Autodesk Fusion 360 part; units mm, degrees
(part 14 of 14)
  line L10014 (-7.2618, 368.3) -> (-12.7611, 377.825)
  line L10015 (-12.7611, 358.775) -> (-7.2618, 368.3)
  line L10016 (6.4863, 388.9375) -> (-4.5122, 388.9375)
  line L10017 (-4.5122, 388.9375) -> (-10.0114, 379.4125)
  line L10018 (-10.0114, 379.4125) -> (-4.5122, 369.8875)
  line L10019 (-4.5122, 369.8875) -> (6.4863, 369.8875)
  line L10020 (11.9856, 379.4125) -> (6.4863, 388.9375)
  line L10021 (6.4863, 369.8875) -> (11.9856, 379.4125)
  line L10022 (25.7337, 400.05) -> (14.7352, 400.05)
  line L10023 (14.7352, 400.05) -> (9.236, 390.525)
  line L10024 (9.236, 390.525) -> (14.7352, 381)
  line L10025 (14.7352, 381) -> (25.7337, 381)
  line L10026 (31.233, 390.525) -> (25.7337, 400.05)
  line L10027 (25.7337, 381) -> (31.233, 390.525)
  line L10028 (44.9812, 411.1625) -> (33.9826, 411.1625)
  line L10029 (33.9826, 411.1625) -> (28.4834, 401.6375)
  line L10030 (28.4834, 401.6375) -> (33.9826, 392.1125)
  line L10031 (33.9826, 392.1125) -> (44.9812, 392.1125)
  line L10032 (50.4804, 401.6375) -> (44.9812, 411.1625)
  line L10033 (44.9812, 392.1125) -> (50.4804, 401.6375)
  line L10034 (64.2286, 422.275) -> (53.2301, 422.275)
  line L10035 (53.2301, 422.275) -> (47.7308, 412.75)
  line L10036 (47.7308, 412.75) -> (53.2301, 403.225)
  line L10037 (53.2301, 403.225) -> (64.2286, 403.225)
  line L10038 (69.7278, 412.75) -> (64.2286, 422.275)
  line L10039 (64.2286, 403.225) -> (69.7278, 412.75)
  line L10040 (83.476, 433.3875) -> (72.4775, 433.3875)
  line L10041 (72.4775, 433.3875) -> (66.9782, 423.8625)
  line L10042 (66.9782, 423.8625) -> (72.4775, 414.3375)
  line L10043 (72.4775, 414.3375) -> (83.476, 414.3375)
  line L10044 (88.9753, 423.8625) -> (83.476, 433.3875)
  line L10045 (83.476, 414.3375) -> (88.9753, 423.8625)
  line L10046 (102.7234, 444.5) -> (91.7249, 444.5)
  line L10047 (91.7249, 444.5) -> (86.2256, 434.975)
  line L10048 (86.2256, 434.975) -> (91.7249, 425.45)
  line L10049 (91.7249, 425.45) -> (102.7234, 425.45)
  line L10050 (108.2227, 434.975) -> (102.7234, 444.5)
  line L10051 (102.7234, 425.45) -> (108.2227, 434.975)
  line L10052 (121.9708, 455.6125) -> (110.9723, 455.6125)
  line L10053 (110.9723, 455.6125) -> (105.473, 446.0875)
  line L10054 (105.473, 446.0875) -> (110.9723, 436.5625)
  line L10055 (110.9723, 436.5625) -> (121.9708, 436.5625)
  line L10056 (127.4701, 446.0875) -> (121.9708, 455.6125)
  line L10057 (121.9708, 436.5625) -> (127.4701, 446.0875)
  line L10058 (141.2182, 466.725) -> (130.2197, 466.725)
  line L10059 (130.2197, 466.725) -> (124.7205, 457.2)
  line L10060 (124.7205, 457.2) -> (130.2197, 447.675)
  line L10061 (130.2197, 447.675) -> (141.2182, 447.675)
  line L10062 (146.7175, 457.2) -> (141.2182, 466.725)
  line L10063 (141.2182, 447.675) -> (146.7175, 457.2)
  line L10064 (160.4657, 477.8375) -> (149.4671, 477.8375)
  line L10065 (149.4671, 477.8375) -> (143.9679, 468.3125)
  line L10066 (143.9679, 468.3125) -> (149.4671, 458.7875)
  line L10067 (149.4671, 458.7875) -> (160.4657, 458.7875)
  line L10068 (165.9649, 468.3125) -> (160.4657, 477.8375)
  line L10069 (160.4657, 458.7875) -> (165.9649, 468.3125)
  line L10070 (179.7131, 488.95) -> (168.7145, 488.95)
  line L10071 (168.7145, 488.95) -> (163.2153, 479.425)
  line L10072 (163.2153, 479.425) -> (168.7145, 469.9)
  line L10073 (168.7145, 469.9) -> (179.7131, 469.9)
  line L10074 (185.2123, 479.425) -> (179.7131, 488.95)
  line L10075 (179.7131, 469.9) -> (185.2123, 479.425)
  line L10076 (198.9605, 500.0625) -> (187.962, 500.0625)
  line L10077 (187.962, 500.0625) -> (182.4627, 490.5375)
  line L10078 (182.4627, 490.5375) -> (187.962, 481.0125)
  line L10079 (187.962, 481.0125) -> (198.9605, 481.0125)
  line L10080 (204.4597, 490.5375) -> (198.9605, 500.0625)
  line L10081 (198.9605, 481.0125) -> (204.4597, 490.5375)
  line L10082 (218.2079, 511.175) -> (207.2094, 511.175)
  line L10083 (207.2094, 511.175) -> (201.7101, 501.65)
  line L10084 (201.7101, 501.65) -> (207.2094, 492.125)
  line L10085 (207.2094, 492.125) -> (218.2079, 492.125)
  line L10086 (223.7072, 501.65) -> (218.2079, 511.175)
  line L10087 (218.2079, 492.125) -> (223.7072, 501.65)
  line L10088 (237.4553, 522.2875) -> (226.4568, 522.2875)
  line L10089 (226.4568, 522.2875) -> (220.9575, 512.7625)
  line L10090 (220.9575, 512.7625) -> (226.4568, 503.2375)
  line L10091 (226.4568, 503.2375) -> (237.4553, 503.2375)
  line L10092 (242.9546, 512.7625) -> (237.4553, 522.2875)
  line L10093 (237.4553, 503.2375) -> (242.9546, 512.7625)
  line L10094 (-917.3896, -122.2375) -> (-928.3881, -122.2375)
  line L10095 (-928.3881, -122.2375) -> (-933.8874, -131.7625)
  line L10096 (-933.8874, -131.7625) -> (-928.3881, -141.2875)
  line L10097 (-928.3881, -141.2875) -> (-917.3896, -141.2875)
  line L10098 (-911.8903, -131.7625) -> (-917.3896, -122.2375)
  line L10099 (-917.3896, -141.2875) -> (-911.8903, -131.7625)
  line L10100 (-898.1422, -111.125) -> (-909.1407, -111.125)
  line L10101 (-909.1407, -111.125) -> (-914.6399, -120.65)
  line L10102 (-914.6399, -120.65) -> (-909.1407, -130.175)
  line L10103 (-909.1407, -130.175) -> (-898.1422, -130.175)
  line L10104 (-892.6429, -120.65) -> (-898.1422, -111.125)
  line L10105 (-898.1422, -130.175) -> (-892.6429, -120.65)
  line L10106 (-878.8947, -100.0125) -> (-889.8933, -100.0125)
  line L10107 (-889.8933, -100.0125) -> (-895.3925, -109.5375)
  line L10108 (-895.3925, -109.5375) -> (-889.8933, -119.0625)
  line L10109 (-889.8933, -119.0625) -> (-878.8947, -119.0625)
  line L10110 (-873.3955, -109.5375) -> (-878.8947, -100.0125)
  line L10111 (-878.8947, -119.0625) -> (-873.3955, -109.5375)
  line L10112 (-859.6473, -88.9) -> (-870.6458, -88.9)
  line L10113 (-870.6458, -88.9) -> (-876.1451, -98.425)
  line L10114 (-876.1451, -98.425) -> (-870.6458, -107.95)
  line L10115 (-870.6458, -107.95) -> (-859.6473, -107.95)
  line L10116 (-854.1481, -98.425) -> (-859.6473, -88.9)
  line L10117 (-859.6473, -107.95) -> (-854.1481, -98.425)
  line L10118 (-840.3999, -77.7875) -> (-851.3984, -77.7875)
  line L10119 (-851.3984, -77.7875) -> (-856.8977, -87.3125)
  line L10120 (-856.8977, -87.3125) -> (-851.3984, -96.8375)
  line L10121 (-851.3984, -96.8375) -> (-840.3999, -96.8375)
  line L10122 (-834.9006, -87.3125) -> (-840.3999, -77.7875)
  line L10123 (-840.3999, -96.8375) -> (-834.9006, -87.3125)
  line L10124 (-821.1525, -66.675) -> (-832.151, -66.675)
  line L10125 (-832.151, -66.675) -> (-837.6503, -76.2)
  line L10126 (-837.6503, -76.2) -> (-832.151, -85.725)
  line L10127 (-832.151, -85.725) -> (-821.1525, -85.725)
  line L10128 (-815.6532, -76.2) -> (-821.1525, -66.675)
  line L10129 (-821.1525, -85.725) -> (-815.6532, -76.2)
  line L10130 (-801.9051, -55.5625) -> (-812.9036, -55.5625)
  line L10131 (-812.9036, -55.5625) -> (-818.4029, -65.0875)
  line L10132 (-818.4029, -65.0875) -> (-812.9036, -74.6125)
  line L10133 (-812.9036, -74.6125) -> (-801.9051, -74.6125)
  line L10134 (-796.4058, -65.0875) -> (-801.9051, -55.5625)
  line L10135 (-801.9051, -74.6125) -> (-796.4058, -65.0875)
  line L10136 (-782.6577, -44.45) -> (-793.6562, -44.45)
  line L10137 (-793.6562, -44.45) -> (-799.1554, -53.975)
  line L10138 (-799.1554, -53.975) -> (-793.6562, -63.5)
  line L10139 (-793.6562, -63.5) -> (-782.6577, -63.5)
  line L10140 (-777.1584, -53.975) -> (-782.6577, -44.45)
  line L10141 (-782.6577, -63.5) -> (-777.1584, -53.975)
  line L10142 (-763.4102, -33.3375) -> (-774.4088, -33.3375)
  line L10143 (-774.4088, -33.3375) -> (-779.908, -42.8625)
  line L10144 (-779.908, -42.8625) -> (-774.4088, -52.3875)
  line L10145 (-774.4088, -52.3875) -> (-763.4102, -52.3875)
  line L10146 (-757.911, -42.8625) -> (-763.4102, -33.3375)
  line L10147 (-763.4102, -52.3875) -> (-757.911, -42.8625)
  line L10148 (-744.1628, -22.225) -> (-755.1614, -22.225)
  line L10149 (-755.1614, -22.225) -> (-760.6606, -31.75)
  line L10150 (-760.6606, -31.75) -> (-755.1614, -41.275)
  line L10151 (-755.1614, -41.275) -> (-744.1628, -41.275)
  line L10152 (-738.6636, -31.75) -> (-744.1628, -22.225)
  line L10153 (-744.1628, -41.275) -> (-738.6636, -31.75)
  line L10154 (-724.9154, -11.1125) -> (-735.9139, -11.1125)
  line L10155 (-735.9139, -11.1125) -> (-741.4132, -20.6375)
  line L10156 (-741.4132, -20.6375) -> (-735.9139, -30.1625)
  line L10157 (-735.9139, -30.1625) -> (-724.9154, -30.1625)
  line L10158 (-719.4162, -20.6375) -> (-724.9154, -11.1125)
  line L10159 (-724.9154, -30.1625) -> (-719.4162, -20.6375)
  line L10160 (-705.668, 0) -> (-716.6665, 0)
  line L10161 (-716.6665, 0) -> (-722.1658, -9.525)
  line L10162 (-722.1658, -9.525) -> (-716.6665, -19.05)
  line L10163 (-716.6665, -19.05) -> (-705.668, -19.05)
  line L10164 (-700.1687, -9.525) -> (-705.668, 0)
  line L10165 (-705.668, -19.05) -> (-700.1687, -9.525)
  line L10166 (-686.4206, 11.1125) -> (-697.4191, 11.1125)
  line L10167 (-697.4191, 11.1125) -> (-702.9184, 1.5875)
  line L10168 (-702.9184, 1.5875) -> (-697.4191, -7.9375)
  line L10169 (-697.4191, -7.9375) -> (-686.4206, -7.9375)
  line L10170 (-680.9213, 1.5875) -> (-686.4206, 11.1125)
  line L10171 (-686.4206, -7.9375) -> (-680.9213, 1.5875)
  line L10172 (-667.1732, 22.225) -> (-678.1717, 22.225)
  line L10173 (-678.1717, 22.225) -> (-683.671, 12.7)
  line L10174 (-683.671, 12.7) -> (-678.1717, 3.175)
  line L10175 (-678.1717, 3.175) -> (-667.1732, 3.175)
  line L10176 (-661.6739, 12.7) -> (-667.1732, 22.225)
  line L10177 (-667.1732, 3.175) -> (-661.6739, 12.7)
  line L10178 (-647.9258, 33.3375) -> (-658.9243, 33.3375)
  line L10179 (-658.9243, 33.3375) -> (-664.4235, 23.8125)
  line L10180 (-664.4235, 23.8125) -> (-658.9243, 14.2875)
  line L10181 (-658.9243, 14.2875) -> (-647.9258, 14.2875)
  line L10182 (-642.4265, 23.8125) -> (-647.9258, 33.3375)
  line L10183 (-647.9258, 14.2875) -> (-642.4265, 23.8125)
  line L10184 (-628.6783, 44.45) -> (-639.6769, 44.45)
  line L10185 (-639.6769, 44.45) -> (-645.1761, 34.925)
  line L10186 (-645.1761, 34.925) -> (-639.6769, 25.4)
  line L10187 (-639.6769, 25.4) -> (-628.6783, 25.4)
  line L10188 (-623.1791, 34.925) -> (-628.6783, 44.45)
  line L10189 (-628.6783, 25.4) -> (-623.1791, 34.925)
  line L10190 (-609.4309, 55.5625) -> (-620.4295, 55.5625)
  line L10191 (-620.4295, 55.5625) -> (-625.9287, 46.0375)
  line L10192 (-625.9287, 46.0375) -> (-620.4295, 36.5125)
  line L10193 (-620.4295, 36.5125) -> (-609.4309, 36.5125)
  line L10194 (-603.9317, 46.0375) -> (-609.4309, 55.5625)
  line L10195 (-609.4309, 36.5125) -> (-603.9317, 46.0375)
  line L10196 (-590.1835, 66.675) -> (-601.182, 66.675)
  line L10197 (-601.182, 66.675) -> (-606.6813, 57.15)
  line L10198 (-606.6813, 57.15) -> (-601.182, 47.625)
  line L10199 (-601.182, 47.625) -> (-590.1835, 47.625)
  line L10200 (-584.6843, 57.15) -> (-590.1835, 66.675)
  line L10201 (-590.1835, 47.625) -> (-584.6843, 57.15)
  line L10202 (-570.9361, 77.7875) -> (-581.9346, 77.7875)
  line L10203 (-581.9346, 77.7875) -> (-587.4339, 68.2625)
  line L10204 (-587.4339, 68.2625) -> (-581.9346, 58.7375)
  line L10205 (-581.9346, 58.7375) -> (-570.9361, 58.7375)
  line L10206 (-565.4368, 68.2625) -> (-570.9361, 77.7875)
  line L10207 (-570.9361, 58.7375) -> (-565.4368, 68.2625)
  line L10208 (-551.6887, 88.9) -> (-562.6872, 88.9)
  line L10209 (-562.6872, 88.9) -> (-568.1865, 79.375)
  line L10210 (-568.1865, 79.375) -> (-562.6872, 69.85)
  line L10211 (-562.6872, 69.85) -> (-551.6887, 69.85)
  line L10212 (-546.1894, 79.375) -> (-551.6887, 88.9)
  line L10213 (-551.6887, 69.85) -> (-546.1894, 79.375)
  line L10214 (-532.4413, 100.0125) -> (-543.4398, 100.0125)
  line L10215 (-543.4398, 100.0125) -> (-548.9391, 90.4875)
  line L10216 (-548.9391, 90.4875) -> (-543.4398, 80.9625)
  line L10217 (-543.4398, 80.9625) -> (-532.4413, 80.9625)
  line L10218 (-526.942, 90.4875) -> (-532.4413, 100.0125)
  line L10219 (-532.4413, 80.9625) -> (-526.942, 90.4875)
  line L10220 (-513.1939, 111.125) -> (-524.1924, 111.125)
  line L10221 (-524.1924, 111.125) -> (-529.6916, 101.6)
  line L10222 (-529.6916, 101.6) -> (-524.1924, 92.075)
  line L10223 (-524.1924, 92.075) -> (-513.1939, 92.075)
  line L10224 (-507.6946, 101.6) -> (-513.1939, 111.125)
  line L10225 (-513.1939, 92.075) -> (-507.6946, 101.6)
  line L10226 (-493.9464, 122.2375) -> (-504.945, 122.2375)
  line L10227 (-504.945, 122.2375) -> (-510.4442, 112.7125)
  line L10228 (-510.4442, 112.7125) -> (-504.945, 103.1875)
  line L10229 (-504.945, 103.1875) -> (-493.9464, 103.1875)
  line L10230 (-488.4472, 112.7125) -> (-493.9464, 122.2375)
  line L10231 (-493.9464, 103.1875) -> (-488.4472, 112.7125)
  line L10232 (-474.699, 133.35) -> (-485.6976, 133.35)
  line L10233 (-485.6976, 133.35) -> (-491.1968, 123.825)
  line L10234 (-491.1968, 123.825) -> (-485.6976, 114.3)
  line L10235 (-485.6976, 114.3) -> (-474.699, 114.3)
  line L10236 (-469.1998, 123.825) -> (-474.699, 133.35)
  line L10237 (-474.699, 114.3) -> (-469.1998, 123.825)
  line L10238 (-455.4516, 144.4625) -> (-466.4501, 144.4625)
  line L10239 (-466.4501, 144.4625) -> (-471.9494, 134.9375)
  line L10240 (-471.9494, 134.9375) -> (-466.4501, 125.4125)
  line L10241 (-466.4501, 125.4125) -> (-455.4516, 125.4125)
  line L10242 (-449.9524, 134.9375) -> (-455.4516, 144.4625)
  line L10243 (-455.4516, 125.4125) -> (-449.9524, 134.9375)
  line L10244 (-436.2042, 155.575) -> (-447.2027, 155.575)
  line L10245 (-447.2027, 155.575) -> (-452.702, 146.05)
  line L10246 (-452.702, 146.05) -> (-447.2027, 136.525)
  line L10247 (-447.2027, 136.525) -> (-436.2042, 136.525)
  line L10248 (-430.7049, 146.05) -> (-436.2042, 155.575)
  line L10249 (-436.2042, 136.525) -> (-430.7049, 146.05)
  line L10250 (-416.9568, 166.6875) -> (-427.9553, 166.6875)
  line L10251 (-427.9553, 166.6875) -> (-433.4546, 157.1625)
  line L10252 (-433.4546, 157.1625) -> (-427.9553, 147.6375)
  line L10253 (-427.9553, 147.6375) -> (-416.9568, 147.6375)
  line L10254 (-411.4575, 157.1625) -> (-416.9568, 166.6875)
  line L10255 (-416.9568, 147.6375) -> (-411.4575, 157.1625)
  line L10256 (-397.7094, 177.8) -> (-408.7079, 177.8)
  line L10257 (-408.7079, 177.8) -> (-414.2072, 168.275)
  line L10258 (-414.2072, 168.275) -> (-408.7079, 158.75)
  line L10259 (-408.7079, 158.75) -> (-397.7094, 158.75)
  line L10260 (-392.2101, 168.275) -> (-397.7094, 177.8)
  line L10261 (-397.7094, 158.75) -> (-392.2101, 168.275)
  line L10262 (-378.462, 188.9125) -> (-389.4605, 188.9125)
  line L10263 (-389.4605, 188.9125) -> (-394.9597, 179.3875)
  line L10264 (-394.9597, 179.3875) -> (-389.4605, 169.8625)
  line L10265 (-389.4605, 169.8625) -> (-378.462, 169.8625)
  line L10266 (-372.9627, 179.3875) -> (-378.462, 188.9125)
  line L10267 (-378.462, 169.8625) -> (-372.9627, 179.3875)
  line L10268 (-359.2145, 200.025) -> (-370.2131, 200.025)
  line L10269 (-370.2131, 200.025) -> (-375.7123, 190.5)
  line L10270 (-375.7123, 190.5) -> (-370.2131, 180.975)
  line L10271 (-370.2131, 180.975) -> (-359.2145, 180.975)
  line L10272 (-353.7153, 190.5) -> (-359.2145, 200.025)
  line L10273 (-359.2145, 180.975) -> (-353.7153, 190.5)
  line L10274 (-339.9671, 211.1375) -> (-350.9657, 211.1375)
  line L10275 (-350.9657, 211.1375) -> (-356.4649, 201.6125)
  line L10276 (-356.4649, 201.6125) -> (-350.9657, 192.0875)
  line L10277 (-350.9657, 192.0875) -> (-339.9671, 192.0875)
  line L10278 (-334.4679, 201.6125) -> (-339.9671, 211.1375)
  line L10279 (-339.9671, 192.0875) -> (-334.4679, 201.6125)
  line L10280 (-320.7197, 222.25) -> (-331.7182, 222.25)
  line L10281 (-331.7182, 222.25) -> (-337.2175, 212.725)
  line L10282 (-337.2175, 212.725) -> (-331.7182, 203.2)
  line L10283 (-331.7182, 203.2) -> (-320.7197, 203.2)
  line L10284 (-315.2205, 212.725) -> (-320.7197, 222.25)
  line L10285 (-320.7197, 203.2) -> (-315.2205, 212.725)
  line L10286 (-301.4723, 233.3625) -> (-312.4708, 233.3625)
  line L10287 (-312.4708, 233.3625) -> (-317.9701, 223.8375)
  line L10288 (-317.9701, 223.8375) -> (-312.4708, 214.3125)
  line L10289 (-312.4708, 214.3125) -> (-301.4723, 214.3125)
  line L10290 (-295.973, 223.8375) -> (-301.4723, 233.3625)
  line L10291 (-301.4723, 214.3125) -> (-295.973, 223.8375)
  line L10292 (-282.2249, 244.475) -> (-293.2234, 244.475)
  line L10293 (-293.2234, 244.475) -> (-298.7227, 234.95)
  line L10294 (-298.7227, 234.95) -> (-293.2234, 225.425)
  line L10295 (-293.2234, 225.425) -> (-282.2249, 225.425)
  line L10296 (-276.7256, 234.95) -> (-282.2249, 244.475)
  line L10297 (-282.2249, 225.425) -> (-276.7256, 234.95)
  line L10298 (-262.9775, 255.5875) -> (-273.976, 255.5875)
  line L10299 (-273.976, 255.5875) -> (-279.4753, 246.0625)
  line L10300 (-279.4753, 246.0625) -> (-273.976, 236.5375)
  line L10301 (-273.976, 236.5375) -> (-262.9775, 236.5375)
  line L10302 (-257.4782, 246.0625) -> (-262.9775, 255.5875)
  line L10303 (-262.9775, 236.5375) -> (-257.4782, 246.0625)
  line L10304 (-243.7301, 266.7) -> (-254.7286, 266.7)
  line L10305 (-254.7286, 266.7) -> (-260.2278, 257.175)
  line L10306 (-260.2278, 257.175) -> (-254.7286, 247.65)
  line L10307 (-254.7286, 247.65) -> (-243.7301, 247.65)
  line L10308 (-238.2308, 257.175) -> (-243.7301, 266.7)
  line L10309 (-243.7301, 247.65) -> (-238.2308, 257.175)
  line L10310 (-224.4826, 277.8125) -> (-235.4812, 277.8125)
  line L10311 (-235.4812, 277.8125) -> (-240.9804, 268.2875)
  line L10312 (-240.9804, 268.2875) -> (-235.4812, 258.7625)
  line L10313 (-235.4812, 258.7625) -> (-224.4826, 258.7625)
  line L10314 (-218.9834, 268.2875) -> (-224.4826, 277.8125)
  line L10315 (-224.4826, 258.7625) -> (-218.9834, 268.2875)
  line L10316 (-205.2352, 288.925) -> (-216.2337, 288.925)
  line L10317 (-216.2337, 288.925) -> (-221.733, 279.4)
  line L10318 (-221.733, 279.4) -> (-216.2337, 269.875)
  line L10319 (-216.2337, 269.875) -> (-205.2352, 269.875)
  line L10320 (-199.736, 279.4) -> (-205.2352, 288.925)
  line L10321 (-205.2352, 269.875) -> (-199.736, 279.4)
  line L10322 (-185.9878, 300.0375) -> (-196.9863, 300.0375)
  line L10323 (-196.9863, 300.0375) -> (-202.4856, 290.5125)
  line L10324 (-202.4856, 290.5125) -> (-196.9863, 280.9875)
  line L10325 (-196.9863, 280.9875) -> (-185.9878, 280.9875)
  line L10326 (-180.4886, 290.5125) -> (-185.9878, 300.0375)
  line L10327 (-185.9878, 280.9875) -> (-180.4886, 290.5125)
  line L10328 (-166.7404, 311.15) -> (-177.7389, 311.15)
  line L10329 (-177.7389, 311.15) -> (-183.2382, 301.625)
  line L10330 (-183.2382, 301.625) -> (-177.7389, 292.1)
  line L10331 (-177.7389, 292.1) -> (-166.7404, 292.1)
  line L10332 (-161.2411, 301.625) -> (-166.7404, 311.15)
  line L10333 (-166.7404, 292.1) -> (-161.2411, 301.625)
  line L10334 (-147.493, 322.2625) -> (-158.4915, 322.2625)
  line L10335 (-158.4915, 322.2625) -> (-163.9908, 312.7375)
  line L10336 (-163.9908, 312.7375) -> (-158.4915, 303.2125)
  line L10337 (-158.4915, 303.2125) -> (-147.493, 303.2125)
  line L10338 (-141.9937, 312.7375) -> (-147.493, 322.2625)
  line L10339 (-147.493, 303.2125) -> (-141.9937, 312.7375)
  line L10340 (-128.2456, 333.375) -> (-139.2441, 333.375)
  line L10341 (-139.2441, 333.375) -> (-144.7434, 323.85)
  line L10342 (-144.7434, 323.85) -> (-139.2441, 314.325)
  line L10343 (-139.2441, 314.325) -> (-128.2456, 314.325)
  line L10344 (-122.7463, 323.85) -> (-128.2456, 333.375)
  line L10345 (-128.2456, 314.325) -> (-122.7463, 323.85)
  line L10346 (-108.9982, 344.4875) -> (-119.9967, 344.4875)
  line L10347 (-119.9967, 344.4875) -> (-125.4959, 334.9625)
  line L10348 (-125.4959, 334.9625) -> (-119.9967, 325.4375)
  line L10349 (-119.9967, 325.4375) -> (-108.9982, 325.4375)
  line L10350 (-103.4989, 334.9625) -> (-108.9982, 344.4875)
  line L10351 (-108.9982, 325.4375) -> (-103.4989, 334.9625)
  line L10352 (-89.7507, 355.6) -> (-100.7493, 355.6)
  line L10353 (-100.7493, 355.6) -> (-106.2485, 346.075)
  line L10354 (-106.2485, 346.075) -> (-100.7493, 336.55)
  line L10355 (-100.7493, 336.55) -> (-89.7507, 336.55)
  line L10356 (-84.2515, 346.075) -> (-89.7507, 355.6)
  line L10357 (-89.7507, 336.55) -> (-84.2515, 346.075)
  line L10358 (-70.5033, 366.7125) -> (-81.5018, 366.7125)
  line L10359 (-81.5018, 366.7125) -> (-87.0011, 357.1875)
  line L10360 (-87.0011, 357.1875) -> (-81.5018, 347.6625)
  line L10361 (-81.5018, 347.6625) -> (-70.5033, 347.6625)
  line L10362 (-65.0041, 357.1875) -> (-70.5033, 366.7125)
  line L10363 (-70.5033, 347.6625) -> (-65.0041, 357.1875)
  line L10364 (-51.2559, 377.825) -> (-62.2544, 377.825)
  line L10365 (-62.2544, 377.825) -> (-67.7537, 368.3)
  line L10366 (-67.7537, 368.3) -> (-62.2544, 358.775)
  line L10367 (-62.2544, 358.775) -> (-51.2559, 358.775)
  line L10368 (-45.7566, 368.3) -> (-51.2559, 377.825)
  line L10369 (-51.2559, 358.775) -> (-45.7566, 368.3)
  line L10370 (-32.0085, 388.9375) -> (-43.007, 388.9375)
  line L10371 (-43.007, 388.9375) -> (-48.5063, 379.4125)
  line L10372 (-48.5063, 379.4125) -> (-43.007, 369.8875)
  line L10373 (-43.007, 369.8875) -> (-32.0085, 369.8875)
  line L10374 (-26.5092, 379.4125) -> (-32.0085, 388.9375)
  line L10375 (-32.0085, 369.8875) -> (-26.5092, 379.4125)
  line L10376 (-12.7611, 400.05) -> (-23.7596, 400.05)
  line L10377 (-23.7596, 400.05) -> (-29.2589, 390.525)
  line L10378 (-29.2589, 390.525) -> (-23.7596, 381)
  line L10379 (-23.7596, 381) -> (-12.7611, 381)
  line L10380 (-7.2618, 390.525) -> (-12.7611, 400.05)
  line L10381 (-12.7611, 381) -> (-7.2618, 390.525)
  line L10382 (6.4863, 411.1625) -> (-4.5122, 411.1625)
  line L10383 (-4.5122, 411.1625) -> (-10.0114, 401.6375)
  line L10384 (-10.0114, 401.6375) -> (-4.5122, 392.1125)
  line L10385 (-4.5122, 392.1125) -> (6.4863, 392.1125)
  line L10386 (11.9856, 401.6375) -> (6.4863, 411.1625)
  line L10387 (6.4863, 392.1125) -> (11.9856, 401.6375)
  line L10388 (25.7337, 422.275) -> (14.7352, 422.275)
  line L10389 (14.7352, 422.275) -> (9.236, 412.75)
  line L10390 (9.236, 412.75) -> (14.7352, 403.225)
  line L10391 (14.7352, 403.225) -> (25.7337, 403.225)
  line L10392 (31.233, 412.75) -> (25.7337, 422.275)
  line L10393 (25.7337, 403.225) -> (31.233, 412.75)
  line L10394 (44.9812, 433.3875) -> (33.9826, 433.3875)
  line L10395 (33.9826, 433.3875) -> (28.4834, 423.8625)
  line L10396 (28.4834, 423.8625) -> (33.9826, 414.3375)
  line L10397 (33.9826, 414.3375) -> (44.9812, 414.3375)
  line L10398 (50.4804, 423.8625) -> (44.9812, 433.3875)
  line L10399 (44.9812, 414.3375) -> (50.4804, 423.8625)
  line L10400 (64.2286, 444.5) -> (53.2301, 444.5)
  line L10401 (53.2301, 444.5) -> (47.7308, 434.975)
  line L10402 (47.7308, 434.975) -> (53.2301, 425.45)
  line L10403 (53.2301, 425.45) -> (64.2286, 425.45)
  line L10404 (69.7278, 434.975) -> (64.2286, 444.5)
  line L10405 (64.2286, 425.45) -> (69.7278, 434.975)
  line L10406 (83.476, 455.6125) -> (72.4775, 455.6125)
  line L10407 (72.4775, 455.6125) -> (66.9782, 446.0875)
  line L10408 (66.9782, 446.0875) -> (72.4775, 436.5625)
  line L10409 (72.4775, 436.5625) -> (83.476, 436.5625)
  line L10410 (88.9753, 446.0875) -> (83.476, 455.6125)
  line L10411 (83.476, 436.5625) -> (88.9753, 446.0875)
  line L10412 (102.7234, 466.725) -> (91.7249, 466.725)
  line L10413 (91.7249, 466.725) -> (86.2256, 457.2)
  line L10414 (86.2256, 457.2) -> (91.7249, 447.675)
  line L10415 (91.7249, 447.675) -> (102.7234, 447.675)
  line L10416 (108.2227, 457.2) -> (102.7234, 466.725)
  line L10417 (102.7234, 447.675) -> (108.2227, 457.2)
  line L10418 (121.9708, 477.8375) -> (110.9723, 477.8375)
  line L10419 (110.9723, 477.8375) -> (105.473, 468.3125)
  line L10420 (105.473, 468.3125) -> (110.9723, 458.7875)
  line L10421 (110.9723, 458.7875) -> (121.9708, 458.7875)
  line L10422 (127.4701, 468.3125) -> (121.9708, 477.8375)
  line L10423 (121.9708, 458.7875) -> (127.4701, 468.3125)
  line L10424 (141.2182, 488.95) -> (130.2197, 488.95)
  line L10425 (130.2197, 488.95) -> (124.7205, 479.425)
  line L10426 (124.7205, 479.425) -> (130.2197, 469.9)
  line L10427 (130.2197, 469.9) -> (141.2182, 469.9)
  line L10428 (146.7175, 479.425) -> (141.2182, 488.95)
  line L10429 (141.2182, 469.9) -> (146.7175, 479.425)
  line L10430 (160.4657, 500.0625) -> (149.4671, 500.0625)
  line L10431 (149.4671, 500.0625) -> (143.9679, 490.5375)
  line L10432 (143.9679, 490.5375) -> (149.4671, 481.0125)
  line L10433 (149.4671, 481.0125) -> (160.4657, 481.0125)
  line L10434 (165.9649, 490.5375) -> (160.4657, 500.0625)
  line L10435 (160.4657, 481.0125) -> (165.9649, 490.5375)
  line L10436 (179.7131, 511.175) -> (168.7145, 511.175)
  line L10437 (168.7145, 511.175) -> (163.2153, 501.65)
  line L10438 (163.2153, 501.65) -> (168.7145, 492.125)
  line L10439 (168.7145, 492.125) -> (179.7131, 492.125)
  line L10440 (185.2123, 501.65) -> (179.7131, 511.175)
  line L10441 (179.7131, 492.125) -> (185.2123, 501.65)
  line L10442 (198.9605, 522.2875) -> (187.962, 522.2875)
  line L10443 (187.962, 522.2875) -> (182.4627, 512.7625)
  line L10444 (182.4627, 512.7625) -> (187.962, 503.2375)
  line L10445 (187.962, 503.2375) -> (198.9605, 503.2375)
  line L10446 (204.4597, 512.7625) -> (198.9605, 522.2875)
  line L10447 (198.9605, 503.2375) -> (204.4597, 512.7625)
  line L10448 (218.2079, 533.4) -> (207.2094, 533.4)
  line L10449 (207.2094, 533.4) -> (201.7101, 523.875)
  line L10450 (201.7101, 523.875) -> (207.2094, 514.35)
  line L10451 (207.2094, 514.35) -> (218.2079, 514.35)
  line L10452 (223.7072, 523.875) -> (218.2079, 533.4)
  line L10453 (218.2079, 514.35) -> (223.7072, 523.875)
  line L10454 (-936.637, -111.125) -> (-947.6355, -111.125)
  line L10455 (-947.6355, -111.125) -> (-953.1348, -120.65)
  line L10456 (-953.1348, -120.65) -> (-947.6355, -130.175)
  line L10457 (-947.6355, -130.175) -> (-936.637, -130.175)
  line L10458 (-931.1377, -120.65) -> (-936.637, -111.125)
  line L10459 (-936.637, -130.175) -> (-931.1377, -120.65)
  line L10460 (-917.3896, -100.0125) -> (-928.3881, -100.0125)
  line L10461 (-928.3881, -100.0125) -> (-933.8874, -109.5375)
  line L10462 (-933.8874, -109.5375) -> (-928.3881, -119.0625)
  line L10463 (-928.3881, -119.0625) -> (-917.3896, -119.0625)
  line L10464 (-911.8903, -109.5375) -> (-917.3896, -100.0125)
  line L10465 (-917.3896, -119.0625) -> (-911.8903, -109.5375)
  line L10466 (-898.1422, -88.9) -> (-909.1407, -88.9)
  line L10467 (-909.1407, -88.9) -> (-914.6399, -98.425)
  line L10468 (-914.6399, -98.425) -> (-909.1407, -107.95)
  line L10469 (-909.1407, -107.95) -> (-898.1422, -107.95)
  line L10470 (-892.6429, -98.425) -> (-898.1422, -88.9)
  line L10471 (-898.1422, -107.95) -> (-892.6429, -98.425)
  line L10472 (-878.8947, -77.7875) -> (-889.8933, -77.7875)
  line L10473 (-889.8933, -77.7875) -> (-895.3925, -87.3125)
  line L10474 (-895.3925, -87.3125) -> (-889.8933, -96.8375)
  line L10475 (-889.8933, -96.8375) -> (-878.8947, -96.8375)
  line L10476 (-873.3955, -87.3125) -> (-878.8947, -77.7875)
  line L10477 (-878.8947, -96.8375) -> (-873.3955, -87.3125)
  line L10478 (-859.6473, -66.675) -> (-870.6458, -66.675)
  line L10479 (-870.6458, -66.675) -> (-876.1451, -76.2)
  line L10480 (-876.1451, -76.2) -> (-870.6458, -85.725)
  line L10481 (-870.6458, -85.725) -> (-859.6473, -85.725)
  line L10482 (-854.1481, -76.2) -> (-859.6473, -66.675)
  line L10483 (-859.6473, -85.725) -> (-854.1481, -76.2)
  line L10484 (-840.3999, -55.5625) -> (-851.3984, -55.5625)
  line L10485 (-851.3984, -55.5625) -> (-856.8977, -65.0875)
  line L10486 (-856.8977, -65.0875) -> (-851.3984, -74.6125)
  line L10487 (-851.3984, -74.6125) -> (-840.3999, -74.6125)
  line L10488 (-834.9006, -65.0875) -> (-840.3999, -55.5625)
  line L10489 (-840.3999, -74.6125) -> (-834.9006, -65.0875)
  line L10490 (-821.1525, -44.45) -> (-832.151, -44.45)
  line L10491 (-832.151, -44.45) -> (-837.6503, -53.975)
  line L10492 (-837.6503, -53.975) -> (-832.151, -63.5)
  line L10493 (-832.151, -63.5) -> (-821.1525, -63.5)
  line L10494 (-815.6532, -53.975) -> (-821.1525, -44.45)
  line L10495 (-821.1525, -63.5) -> (-815.6532, -53.975)
  line L10496 (-801.9051, -33.3375) -> (-812.9036, -33.3375)
  line L10497 (-812.9036, -33.3375) -> (-818.4029, -42.8625)
  line L10498 (-818.4029, -42.8625) -> (-812.9036, -52.3875)
  line L10499 (-812.9036, -52.3875) -> (-801.9051, -52.3875)
  line L10500 (-796.4058, -42.8625) -> (-801.9051, -33.3375)
  line L10501 (-801.9051, -52.3875) -> (-796.4058, -42.8625)
  line L10502 (-782.6577, -22.225) -> (-793.6562, -22.225)
  line L10503 (-793.6562, -22.225) -> (-799.1554, -31.75)
  line L10504 (-799.1554, -31.75) -> (-793.6562, -41.275)
  line L10505 (-793.6562, -41.275) -> (-782.6577, -41.275)
  line L10506 (-777.1584, -31.75) -> (-782.6577, -22.225)
  line L10507 (-782.6577, -41.275) -> (-777.1584, -31.75)
  line L10508 (-763.4102, -11.1125) -> (-774.4088, -11.1125)
  line L10509 (-774.4088, -11.1125) -> (-779.908, -20.6375)
  line L10510 (-779.908, -20.6375) -> (-774.4088, -30.1625)
  line L10511 (-774.4088, -30.1625) -> (-763.4102, -30.1625)
  line L10512 (-757.911, -20.6375) -> (-763.4102, -11.1125)
  line L10513 (-763.4102, -30.1625) -> (-757.911, -20.6375)
  line L10514 (-744.1628, 0) -> (-755.1614, 0)
  line L10515 (-755.1614, 0) -> (-760.6606, -9.525)
  line L10516 (-760.6606, -9.525) -> (-755.1614, -19.05)
  line L10517 (-755.1614, -19.05) -> (-744.1628, -19.05)
  line L10518 (-738.6636, -9.525) -> (-744.1628, 0)
  line L10519 (-744.1628, -19.05) -> (-738.6636, -9.525)
  line L10520 (-724.9154, 11.1125) -> (-735.9139, 11.1125)
  line L10521 (-735.9139, 11.1125) -> (-741.4132, 1.5875)
  line L10522 (-741.4132, 1.5875) -> (-735.9139, -7.9375)
  line L10523 (-735.9139, -7.9375) -> (-724.9154, -7.9375)
  line L10524 (-719.4162, 1.5875) -> (-724.9154, 11.1125)
  line L10525 (-724.9154, -7.9375) -> (-719.4162, 1.5875)
  line L10526 (-705.668, 22.225) -> (-716.6665, 22.225)
  line L10527 (-716.6665, 22.225) -> (-722.1658, 12.7)
  line L10528 (-722.1658, 12.7) -> (-716.6665, 3.175)
  line L10529 (-716.6665, 3.175) -> (-705.668, 3.175)
  line L10530 (-700.1687, 12.7) -> (-705.668, 22.225)
  line L10531 (-705.668, 3.175) -> (-700.1687, 12.7)
  line L10532 (-686.4206, 33.3375) -> (-697.4191, 33.3375)
  line L10533 (-697.4191, 33.3375) -> (-702.9184, 23.8125)
  line L10534 (-702.9184, 23.8125) -> (-697.4191, 14.2875)
  line L10535 (-697.4191, 14.2875) -> (-686.4206, 14.2875)
  line L10536 (-680.9213, 23.8125) -> (-686.4206, 33.3375)
  line L10537 (-686.4206, 14.2875) -> (-680.9213, 23.8125)
  line L10538 (-667.1732, 44.45) -> (-678.1717, 44.45)
  line L10539 (-678.1717, 44.45) -> (-683.671, 34.925)
  line L10540 (-683.671, 34.925) -> (-678.1717, 25.4)
  line L10541 (-678.1717, 25.4) -> (-667.1732, 25.4)
  line L10542 (-661.6739, 34.925) -> (-667.1732, 44.45)
  line L10543 (-667.1732, 25.4) -> (-661.6739, 34.925)
  line L10544 (-647.9258, 55.5625) -> (-658.9243, 55.5625)
  line L10545 (-658.9243, 55.5625) -> (-664.4235, 46.0375)
  line L10546 (-664.4235, 46.0375) -> (-658.9243, 36.5125)
  line L10547 (-658.9243, 36.5125) -> (-647.9258, 36.5125)
  line L10548 (-642.4265, 46.0375) -> (-647.9258, 55.5625)
  line L10549 (-647.9258, 36.5125) -> (-642.4265, 46.0375)
  line L10550 (-628.6783, 66.675) -> (-639.6769, 66.675)
  line L10551 (-639.6769, 66.675) -> (-645.1761, 57.15)
  line L10552 (-645.1761, 57.15) -> (-639.6769, 47.625)
  line L10553 (-639.6769, 47.625) -> (-628.6783, 47.625)
  line L10554 (-623.1791, 57.15) -> (-628.6783, 66.675)
  line L10555 (-628.6783, 47.625) -> (-623.1791, 57.15)
  line L10556 (-609.4309, 77.7875) -> (-620.4295, 77.7875)
  line L10557 (-620.4295, 77.7875) -> (-625.9287, 68.2625)
  line L10558 (-625.9287, 68.2625) -> (-620.4295, 58.7375)
  line L10559 (-620.4295, 58.7375) -> (-609.4309, 58.7375)
  line L10560 (-603.9317, 68.2625) -> (-609.4309, 77.7875)
  line L10561 (-609.4309, 58.7375) -> (-603.9317, 68.2625)
  line L10562 (-590.1835, 88.9) -> (-601.182, 88.9)
  line L10563 (-601.182, 88.9) -> (-606.6813, 79.375)
  line L10564 (-606.6813, 79.375) -> (-601.182, 69.85)
  line L10565 (-601.182, 69.85) -> (-590.1835, 69.85)
  line L10566 (-584.6843, 79.375) -> (-590.1835, 88.9)
  line L10567 (-590.1835, 69.85) -> (-584.6843, 79.375)
  line L10568 (-570.9361, 100.0125) -> (-581.9346, 100.0125)
  line L10569 (-581.9346, 100.0125) -> (-587.4339, 90.4875)
  line L10570 (-587.4339, 90.4875) -> (-581.9346, 80.9625)
  line L10571 (-581.9346, 80.9625) -> (-570.9361, 80.9625)
  line L10572 (-565.4368, 90.4875) -> (-570.9361, 100.0125)
  line L10573 (-570.9361, 80.9625) -> (-565.4368, 90.4875)
  line L10574 (-551.6887, 111.125) -> (-562.6872, 111.125)
  line L10575 (-562.6872, 111.125) -> (-568.1865, 101.6)
  line L10576 (-568.1865, 101.6) -> (-562.6872, 92.075)
  line L10577 (-562.6872, 92.075) -> (-551.6887, 92.075)
  line L10578 (-546.1894, 101.6) -> (-551.6887, 111.125)
  line L10579 (-551.6887, 92.075) -> (-546.1894, 101.6)
  line L10580 (-532.4413, 122.2375) -> (-543.4398, 122.2375)
  line L10581 (-543.4398, 122.2375) -> (-548.9391, 112.7125)
  line L10582 (-548.9391, 112.7125) -> (-543.4398, 103.1875)
  line L10583 (-543.4398, 103.1875) -> (-532.4413, 103.1875)
  line L10584 (-526.942, 112.7125) -> (-532.4413, 122.2375)
  line L10585 (-532.4413, 103.1875) -> (-526.942, 112.7125)
  line L10586 (-513.1939, 133.35) -> (-524.1924, 133.35)
  line L10587 (-524.1924, 133.35) -> (-529.6916, 123.825)
  line L10588 (-529.6916, 123.825) -> (-524.1924, 114.3)
  line L10589 (-524.1924, 114.3) -> (-513.1939, 114.3)
  line L10590 (-507.6946, 123.825) -> (-513.1939, 133.35)
  line L10591 (-513.1939, 114.3) -> (-507.6946, 123.825)
  line L10592 (-493.9464, 144.4625) -> (-504.945, 144.4625)
  line L10593 (-504.945, 144.4625) -> (-510.4442, 134.9375)
  line L10594 (-510.4442, 134.9375) -> (-504.945, 125.4125)
  line L10595 (-504.945, 125.4125) -> (-493.9464, 125.4125)
  line L10596 (-488.4472, 134.9375) -> (-493.9464, 144.4625)
  line L10597 (-493.9464, 125.4125) -> (-488.4472, 134.9375)
  line L10598 (-474.699, 155.575) -> (-485.6976, 155.575)
  line L10599 (-485.6976, 155.575) -> (-491.1968, 146.05)
  line L10600 (-491.1968, 146.05) -> (-485.6976, 136.525)
  line L10601 (-485.6976, 136.525) -> (-474.699, 136.525)
  line L10602 (-469.1998, 146.05) -> (-474.699, 155.575)
  line L10603 (-474.699, 136.525) -> (-469.1998, 146.05)
  line L10604 (-455.4516, 166.6875) -> (-466.4501, 166.6875)
  line L10605 (-466.4501, 166.6875) -> (-471.9494, 157.1625)
  line L10606 (-471.9494, 157.1625) -> (-466.4501, 147.6375)
  line L10607 (-466.4501, 147.6375) -> (-455.4516, 147.6375)
  line L10608 (-449.9524, 157.1625) -> (-455.4516, 166.6875)
  line L10609 (-455.4516, 147.6375) -> (-449.9524, 157.1625)
  line L10610 (-436.2042, 177.8) -> (-447.2027, 177.8)
  line L10611 (-447.2027, 177.8) -> (-452.702, 168.275)
  line L10612 (-452.702, 168.275) -> (-447.2027, 158.75)
  line L10613 (-447.2027, 158.75) -> (-436.2042, 158.75)
  line L10614 (-430.7049, 168.275) -> (-436.2042, 177.8)
  line L10615 (-436.2042, 158.75) -> (-430.7049, 168.275)
  line L10616 (-416.9568, 188.9125) -> (-427.9553, 188.9125)
  line L10617 (-427.9553, 188.9125) -> (-433.4546, 179.3875)
  line L10618 (-433.4546, 179.3875) -> (-427.9553, 169.8625)
  line L10619 (-427.9553, 169.8625) -> (-416.9568, 169.8625)
  line L10620 (-411.4575, 179.3875) -> (-416.9568, 188.9125)
  line L10621 (-416.9568, 169.8625) -> (-411.4575, 179.3875)
  line L10622 (-397.7094, 200.025) -> (-408.7079, 200.025)
  line L10623 (-408.7079, 200.025) -> (-414.2072, 190.5)
  line L10624 (-414.2072, 190.5) -> (-408.7079, 180.975)
  line L10625 (-408.7079, 180.975) -> (-397.7094, 180.975)
  line L10626 (-392.2101, 190.5) -> (-397.7094, 200.025)
  line L10627 (-397.7094, 180.975) -> (-392.2101, 190.5)
  line L10628 (-378.462, 211.1375) -> (-389.4605, 211.1375)
  line L10629 (-389.4605, 211.1375) -> (-394.9597, 201.6125)
  line L10630 (-394.9597, 201.6125) -> (-389.4605, 192.0875)
  line L10631 (-389.4605, 192.0875) -> (-378.462, 192.0875)
  line L10632 (-372.9627, 201.6125) -> (-378.462, 211.1375)
  line L10633 (-378.462, 192.0875) -> (-372.9627, 201.6125)
  line L10634 (-359.2145, 222.25) -> (-370.2131, 222.25)
  line L10635 (-370.2131, 222.25) -> (-375.7123, 212.725)
  line L10636 (-375.7123, 212.725) -> (-370.2131, 203.2)
  line L10637 (-370.2131, 203.2) -> (-359.2145, 203.2)
  line L10638 (-353.7153, 212.725) -> (-359.2145, 222.25)
  line L10639 (-359.2145, 203.2) -> (-353.7153, 212.725)
  line L10640 (-339.9671, 233.3625) -> (-350.9657, 233.3625)
  line L10641 (-350.9657, 233.3625) -> (-356.4649, 223.8375)
  line L10642 (-356.4649, 223.8375) -> (-350.9657, 214.3125)
  line L10643 (-350.9657, 214.3125) -> (-339.9671, 214.3125)
  line L10644 (-334.4679, 223.8375) -> (-339.9671, 233.3625)
  line L10645 (-339.9671, 214.3125) -> (-334.4679, 223.8375)
  line L10646 (-320.7197, 244.475) -> (-331.7182, 244.475)
  line L10647 (-331.7182, 244.475) -> (-337.2175, 234.95)
  line L10648 (-337.2175, 234.95) -> (-331.7182, 225.425)
  line L10649 (-331.7182, 225.425) -> (-320.7197, 225.425)
  line L10650 (-315.2205, 234.95) -> (-320.7197, 244.475)
  line L10651 (-320.7197, 225.425) -> (-315.2205, 234.95)
  line L10652 (-301.4723, 255.5875) -> (-312.4708, 255.5875)
  line L10653 (-312.4708, 255.5875) -> (-317.9701, 246.0625)
  line L10654 (-317.9701, 246.0625) -> (-312.4708, 236.5375)
  line L10655 (-312.4708, 236.5375) -> (-301.4723, 236.5375)
  line L10656 (-295.973, 246.0625) -> (-301.4723, 255.5875)
  line L10657 (-301.4723, 236.5375) -> (-295.973, 246.0625)
  line L10658 (-282.2249, 266.7) -> (-293.2234, 266.7)
  line L10659 (-293.2234, 266.7) -> (-298.7227, 257.175)
  line L10660 (-298.7227, 257.175) -> (-293.2234, 247.65)
  line L10661 (-293.2234, 247.65) -> (-282.2249, 247.65)
  line L10662 (-276.7256, 257.175) -> (-282.2249, 266.7)
  line L10663 (-282.2249, 247.65) -> (-276.7256, 257.175)
  line L10664 (-262.9775, 277.8125) -> (-273.976, 277.8125)
  line L10665 (-273.976, 277.8125) -> (-279.4753, 268.2875)
  line L10666 (-279.4753, 268.2875) -> (-273.976, 258.7625)
  line L10667 (-273.976, 258.7625) -> (-262.9775, 258.7625)
  line L10668 (-257.4782, 268.2875) -> (-262.9775, 277.8125)
  line L10669 (-262.9775, 258.7625) -> (-257.4782, 268.2875)
  line L10670 (-243.7301, 288.925) -> (-254.7286, 288.925)
  line L10671 (-254.7286, 288.925) -> (-260.2278, 279.4)
  line L10672 (-260.2278, 279.4) -> (-254.7286, 269.875)
  line L10673 (-254.7286, 269.875) -> (-243.7301, 269.875)
  line L10674 (-238.2308, 279.4) -> (-243.7301, 288.925)
  line L10675 (-243.7301, 269.875) -> (-238.2308, 279.4)
  line L10676 (-224.4826, 300.0375) -> (-235.4812, 300.0375)
  line L10677 (-235.4812, 300.0375) -> (-240.9804, 290.5125)
  line L10678 (-240.9804, 290.5125) -> (-235.4812, 280.9875)
  line L10679 (-235.4812, 280.9875) -> (-224.4826, 280.9875)
  line L10680 (-218.9834, 290.5125) -> (-224.4826, 300.0375)
  line L10681 (-224.4826, 280.9875) -> (-218.9834, 290.5125)
  line L10682 (-205.2352, 311.15) -> (-216.2337, 311.15)
  line L10683 (-216.2337, 311.15) -> (-221.733, 301.625)
  line L10684 (-221.733, 301.625) -> (-216.2337, 292.1)
  line L10685 (-216.2337, 292.1) -> (-205.2352, 292.1)
  line L10686 (-199.736, 301.625) -> (-205.2352, 311.15)
  line L10687 (-205.2352, 292.1) -> (-199.736, 301.625)
  line L10688 (-185.9878, 322.2625) -> (-196.9863, 322.2625)
  line L10689 (-196.9863, 322.2625) -> (-202.4856, 312.7375)
  line L10690 (-202.4856, 312.7375) -> (-196.9863, 303.2125)
  line L10691 (-196.9863, 303.2125) -> (-185.9878, 303.2125)
  line L10692 (-180.4886, 312.7375) -> (-185.9878, 322.2625)
  line L10693 (-185.9878, 303.2125) -> (-180.4886, 312.7375)
  line L10694 (-166.7404, 333.375) -> (-177.7389, 333.375)
  line L10695 (-177.7389, 333.375) -> (-183.2382, 323.85)
  line L10696 (-183.2382, 323.85) -> (-177.7389, 314.325)
  line L10697 (-177.7389, 314.325) -> (-166.7404, 314.325)
  line L10698 (-161.2411, 323.85) -> (-166.7404, 333.375)
  line L10699 (-166.7404, 314.325) -> (-161.2411, 323.85)
  line L10700 (-147.493, 344.4875) -> (-158.4915, 344.4875)
  line L10701 (-158.4915, 344.4875) -> (-163.9908, 334.9625)
  line L10702 (-163.9908, 334.9625) -> (-158.4915, 325.4375)
  line L10703 (-158.4915, 325.4375) -> (-147.493, 325.4375)
  line L10704 (-141.9937, 334.9625) -> (-147.493, 344.4875)
  line L10705 (-147.493, 325.4375) -> (-141.9937, 334.9625)
  line L10706 (-128.2456, 355.6) -> (-139.2441, 355.6)
  line L10707 (-139.2441, 355.6) -> (-144.7434, 346.075)
  line L10708 (-144.7434, 346.075) -> (-139.2441, 336.55)
  line L10709 (-139.2441, 336.55) -> (-128.2456, 336.55)
  line L10710 (-122.7463, 346.075) -> (-128.2456, 355.6)
  line L10711 (-128.2456, 336.55) -> (-122.7463, 346.075)
  line L10712 (-108.9982, 366.7125) -> (-119.9967, 366.7125)
  line L10713 (-119.9967, 366.7125) -> (-125.4959, 357.1875)
  line L10714 (-125.4959, 357.1875) -> (-119.9967, 347.6625)
  line L10715 (-119.9967, 347.6625) -> (-108.9982, 347.6625)
  line L10716 (-103.4989, 357.1875) -> (-108.9982, 366.7125)
  line L10717 (-108.9982, 347.6625) -> (-103.4989, 357.1875)
  line L10718 (-89.7507, 377.825) -> (-100.7493, 377.825)
  line L10719 (-100.7493, 377.825) -> (-106.2485, 368.3)
  line L10720 (-106.2485, 368.3) -> (-100.7493, 358.775)
  line L10721 (-100.7493, 358.775) -> (-89.7507, 358.775)
  line L10722 (-84.2515, 368.3) -> (-89.7507, 377.825)
  line L10723 (-89.7507, 358.775) -> (-84.2515, 368.3)
  line L10724 (-70.5033, 388.9375) -> (-81.5018, 388.9375)
  line L10725 (-81.5018, 388.9375) -> (-87.0011, 379.4125)
  line L10726 (-87.0011, 379.4125) -> (-81.5018, 369.8875)
  line L10727 (-81.5018, 369.8875) -> (-70.5033, 369.8875)
  line L10728 (-65.0041, 379.4125) -> (-70.5033, 388.9375)
  line L10729 (-70.5033, 369.8875) -> (-65.0041, 379.4125)
  line L10730 (-51.2559, 400.05) -> (-62.2544, 400.05)
  line L10731 (-62.2544, 400.05) -> (-67.7537, 390.525)
  line L10732 (-67.7537, 390.525) -> (-62.2544, 381)
  line L10733 (-62.2544, 381) -> (-51.2559, 381)
  line L10734 (-45.7566, 390.525) -> (-51.2559, 400.05)
  line L10735 (-51.2559, 381) -> (-45.7566, 390.525)
  line L10736 (-32.0085, 411.1625) -> (-43.007, 411.1625)
  line L10737 (-43.007, 411.1625) -> (-48.5063, 401.6375)
  line L10738 (-48.5063, 401.6375) -> (-43.007, 392.1125)
  line L10739 (-43.007, 392.1125) -> (-32.0085, 392.1125)
  line L10740 (-26.5092, 401.6375) -> (-32.0085, 411.1625)
  line L10741 (-32.0085, 392.1125) -> (-26.5092, 401.6375)
  line L10742 (-12.7611, 422.275) -> (-23.7596, 422.275)
  line L10743 (-23.7596, 422.275) -> (-29.2589, 412.75)
  line L10744 (-29.2589, 412.75) -> (-23.7596, 403.225)
  line L10745 (-23.7596, 403.225) -> (-12.7611, 403.225)
  line L10746 (-7.2618, 412.75) -> (-12.7611, 422.275)
  line L10747 (-12.7611, 403.225) -> (-7.2618, 412.75)
  line L10748 (6.4863, 433.3875) -> (-4.5122, 433.3875)
  line L10749 (-4.5122, 433.3875) -> (-10.0114, 423.8625)
  line L10750 (-10.0114, 423.8625) -> (-4.5122, 414.3375)
  line L10751 (-4.5122, 414.3375) -> (6.4863, 414.3375)
  line L10752 (11.9856, 423.8625) -> (6.4863, 433.3875)
  line L10753 (6.4863, 414.3375) -> (11.9856, 423.8625)
  line L10754 (25.7337, 444.5) -> (14.7352, 444.5)
  line L10755 (14.7352, 444.5) -> (9.236, 434.975)
  line L10756 (9.236, 434.975) -> (14.7352, 425.45)
  line L10757 (14.7352, 425.45) -> (25.7337, 425.45)
  line L10758 (31.233, 434.975) -> (25.7337, 444.5)
  line L10759 (25.7337, 425.45) -> (31.233, 434.975)
  line L10760 (44.9812, 455.6125) -> (33.9826, 455.6125)
  line L10761 (33.9826, 455.6125) -> (28.4834, 446.0875)
  line L10762 (28.4834, 446.0875) -> (33.9826, 436.5625)
  line L10763 (33.9826, 436.5625) -> (44.9812, 436.5625)
  line L10764 (50.4804, 446.0875) -> (44.9812, 455.6125)
  line L10765 (44.9812, 436.5625) -> (50.4804, 446.0875)
  line L10766 (64.2286, 466.725) -> (53.2301, 466.725)
  line L10767 (53.2301, 466.725) -> (47.7308, 457.2)
  line L10768 (47.7308, 457.2) -> (53.2301, 447.675)
  line L10769 (53.2301, 447.675) -> (64.2286, 447.675)
  line L10770 (69.7278, 457.2) -> (64.2286, 466.725)
  line L10771 (64.2286, 447.675) -> (69.7278, 457.2)
  line L10772 (83.476, 477.8375) -> (72.4775, 477.8375)
  line L10773 (72.4775, 477.8375) -> (66.9782, 468.3125)
  line L10774 (66.9782, 468.3125) -> (72.4775, 458.7875)
  line L10775 (72.4775, 458.7875) -> (83.476, 458.7875)
  line L10776 (88.9753, 468.3125) -> (83.476, 477.8375)
  line L10777 (83.476, 458.7875) -> (88.9753, 468.3125)
  line L10778 (102.7234, 488.95) -> (91.7249, 488.95)
  line L10779 (91.7249, 488.95) -> (86.2256, 479.425)
  line L10780 (86.2256, 479.425) -> (91.7249, 469.9)
  line L10781 (91.7249, 469.9) -> (102.7234, 469.9)
  line L10782 (108.2227, 479.425) -> (102.7234, 488.95)
  line L10783 (102.7234, 469.9) -> (108.2227, 479.425)
  line L10784 (121.9708, 500.0625) -> (110.9723, 500.0625)
  line L10785 (110.9723, 500.0625) -> (105.473, 490.5375)
  line L10786 (105.473, 490.5375) -> (110.9723, 481.0125)
  line L10787 (110.9723, 481.0125) -> (121.9708, 481.0125)
  line L10788 (127.4701, 490.5375) -> (121.9708, 500.0625)
  line L10789 (121.9708, 481.0125) -> (127.4701, 490.5375)
  line L10790 (141.2182, 511.175) -> (130.2197, 511.175)
  line L10791 (130.2197, 511.175) -> (124.7205, 501.65)
  line L10792 (124.7205, 501.65) -> (130.2197, 492.125)
  line L10793 (130.2197, 492.125) -> (141.2182, 492.125)
  line L10794 (146.7175, 501.65) -> (141.2182, 511.175)
  line L10795 (141.2182, 492.125) -> (146.7175, 501.65)
  line L10796 (160.4657, 522.2875) -> (149.4671, 522.2875)
  line L10797 (149.4671, 522.2875) -> (143.9679, 512.7625)
  line L10798 (143.9679, 512.7625) -> (149.4671, 503.2375)
  line L10799 (149.4671, 503.2375) -> (160.4657, 503.2375)
  line L10800 (165.9649, 512.7625) -> (160.4657, 522.2875)
  line L10801 (160.4657, 503.2375) -> (165.9649, 512.7625)
  line L10802 (179.7131, 533.4) -> (168.7145, 533.4)
  line L10803 (168.7145, 533.4) -> (163.2153, 523.875)
  line L10804 (163.2153, 523.875) -> (168.7145, 514.35)
  line L10805 (168.7145, 514.35) -> (179.7131, 514.35)
  line L10806 (185.2123, 523.875) -> (179.7131, 533.4)
  line L10807 (179.7131, 514.35) -> (185.2123, 523.875)
  line L10808 (198.9605, 544.5125) -> (187.962, 544.5125)
  line L10809 (187.962, 544.5125) -> (182.4627, 534.9875)
  line L10810 (182.4627, 534.9875) -> (187.962, 525.4625)
  line L10811 (187.962, 525.4625) -> (198.9605, 525.4625)
  line L10812 (204.4597, 534.9875) -> (198.9605, 544.5125)
  line L10813 (198.9605, 525.4625) -> (204.4597, 534.9875)
  line L10814 (413.0575, -142.0113) -> (1204.0643, -142.0113) construction
  line L10815 (1204.0643, -142.0113) -> (1204.0643, -269.0755) construction
  line L10816 (1204.0643, -269.0755) -> (413.0575, -269.0755) construction
  line L10817 (413.0575, -269.0755) -> (413.0575, -142.0113) construction
  point P0 (-95.25, 34.925)
  dimension "d23" = 120
  dimension "d24" = 9.525
  dimension "d27" = 22.225
  dimension "d28" = 22.225
  dimension "d29" = 791.0068
  constraint coincident L5.start L6.start
  constraint coincident L0.start L2.start
  constraint coincident L2.end L3.end
  constraint coincident L6.end L7.end
  constraint horizontal L11
  constraint midpoint L8 P0
  constraint coincident L1 L10.end
  constraint coincident P0 L10.start
  constraint coincident L10 L12.start
  constraint midpoint L17 L18.end
  constraint midpoint L13 L19.end
  constraint horizontal L10814
  constraint vertical L10815
  constraint horizontal L10816
  constraint vertical L10817
  measures "d23" angle of L10 L11
  measures "d24" distance of P0 L17
  measures "d29" distance of L10814.start L10814.end
equation "d8 = ( 3 / 8 ) * 1 in"
equation "d13 = ( 7 / 8 ) * 1 in"
equation "d14 = ( 7 / 8 ) * 1 in"
equation "d24 = ( 3 / 8 ) * 1 in"
equation "d27 = ( 7 / 8 ) * 1 in"
equation "d28 = ( 7 / 8 ) * 1 in"
equation "d29 = 28 in + 3.142 in"
